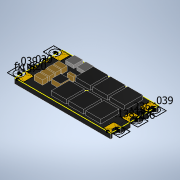
# Autodesk Inventor part: Circuit Board
Saved by Autodesk Inventor 2022 (Build 260153000, 153)
## iProperties
Created: 2022-09-18
Part Number: Circuit Board
Material: PPS Plastic
Document SubType Name: Modeling
Designer: Nathan Cai
Density: 1.637 g/cm^3
Appearance: Smooth - Black
Author: Nathan Cai
Autodesk Inventor part; units mm, degrees
ref_plane "YZ Plane" through (0, 0, 0) normal (1, 0, 0) x (0, 1, 0)
ref_plane "XZ Plane" through (0, 0, 0) normal (0, 1, 0) x (-1, 0, 0)
ref_plane "XY Plane" through (0, 0, 0) normal (0, 0, 1) x (1, 0, 0)
sketch "Sketch1" plane through (0, 0, 0) normal (0, 1, 0) x (-1, 0, 0)
  line L0 (-16, 8) -> (16, 8)
  line L1 (16, 8) -> (16, -8)
  line L2 (16, -8) -> (-16, -8)
  line L3 (-16, -8) -> (-16, 8)
  line L4 (-16, 8) -> (16, -8) construction
  line L5 (16, 8) -> (-16, -8) construction
  point P0 (0, 0)
  dimension "d0" = 32
  dimension "d1" = 16
  constraints: 12 end point, 2 midpoint, 2 parallel, 1 horizontal, 1 perpendicular
  measures "d0" distance of L1.end L2.end
  measures "d1" distance of L0.end L1.end
extrude "Extrusion1" add sketch "Sketch1" along normal blind 0.875
sketch "Sketch2" plane through (0, 0.875, 0) normal (0, 1, 0) x (1, 0, 0)
  line L0 (15, -8.0096) -> (15, 8) construction
  line L1 (16, 8) -> (-16, 8) projected
  line L2 (16, -8) -> (16, 8) projected
  circle A0 centre (16.5, 0) radius 1.5
  line L3 (-16, 8) -> (-16, -8) projected
  line L4 (-16, 0) -> (16, 0) construction
  circle A1 centre (16.5, 6) radius 1.5
  line L5 (18.75, -1.75) -> (13.25, -1.75)
  line L6 (13.25, -1.75) -> (13.25, 1.75)
  line L7 (13.25, 1.75) -> (18.75, 1.75)
  line L8 (18.75, 1.75) -> (18.75, -1.75)
  line L9 (18.75, -1.75) -> (13.25, 1.75) construction
  line L10 (13.25, -1.75) -> (18.75, 1.75) construction
  line L11 (13.25, 4.25) -> (13.25, 7.75)
  line L12 (18.75, 4.25) -> (13.25, 4.25)
  line L13 (18.75, 7.75) -> (18.75, 4.25)
  line L14 (18.75, 4.25) -> (13.25, 7.75) construction
  line L15 (13.25, 4.25) -> (18.75, 7.75) construction
  line L16 (13.25, 7.75) -> (18.75, 7.75)
  circle A2 centre (16.5, -6) radius 1.5
  line L17 (13.25, -4.25) -> (13.25, -7.75)
  line L18 (18.75, -4.25) -> (13.25, -4.25)
  line L19 (18.75, -7.75) -> (18.75, -4.25)
  line L20 (18.75, -4.25) -> (13.25, -7.75) construction
  line L21 (13.25, -4.25) -> (18.75, -7.75) construction
  line L22 (13.25, -7.75) -> (18.75, -7.75)
  line L23 (-16, -8) -> (16, -8) projected
  line L24 (0, -8) -> (0, 8) construction
  line L25 (-15, -8.0096) -> (-15, 8) construction
  circle A3 centre (-16.5, 6) radius 1.5
  line L26 (-13.25, 4.25) -> (-13.25, 7.75)
  line L27 (-18.75, 4.25) -> (-13.25, 4.25)
  line L28 (-18.75, 7.75) -> (-18.75, 4.25)
  line L29 (-18.75, 4.25) -> (-13.25, 7.75) construction
  line L30 (-13.25, 4.25) -> (-18.75, 7.75) construction
  line L31 (-13.25, 7.75) -> (-18.75, 7.75)
  line L32 (-13.25, -4.25) -> (-13.25, -7.75)
  line L33 (-18.75, -4.25) -> (-13.25, -4.25)
  line L34 (-18.75, -4.25) -> (-13.25, -7.75) construction
  line L35 (-13.25, -4.25) -> (-18.75, -7.75) construction
  line L36 (-13.25, -7.75) -> (-18.75, -7.75)
  line L37 (-18.75, -7.75) -> (-18.75, -4.25)
  circle A4 centre (-16.5, -6) radius 1.5
  circle A5 centre (-16, -2) radius 0.5
  circle A6 centre (-16, 2) radius 0.5
  circle A7 centre (-16, -2) radius 1
  circle A8 centre (-16, 2) radius 1
  point P0 (0, 0)
  point P1 (16, 6)
  point P2 (15, -8)
  point P3 (16, -6)
  point P4 (-16, 6)
  point P5 (-15, -8)
  point P6 (-16, -6)
  point P7 (-16, 4.5858)
  point P8 (-16, 7.4142)
  point P9 (16, 4.25)
  point P10 (16, 4.5858)
  point P11 (16, 7.4142)
  point P12 (16, 7.75)
  point P13 (16, -1.75)
  point P14 (16, -1.4142)
  point P15 (16, 1.4142)
  point P16 (16, 1.75)
  point P17 (16, -7.75)
  point P18 (16, -7.4142)
  point P19 (16, -4.5858)
  point P20 (16, -4.25)
  point P21 (-16, 7.75)
  point P22 (-16, 4.25)
  point P23 (-16, -4.25)
  point P24 (-16, -4.5858)
  point P25 (-16, -7.4142)
  point P26 (-16, -7.75)
  point P27 (-16, 3)
  point P28 (-16, 2.5)
  point P29 (-16, 1.5)
  point P30 (-16, 1)
  point P31 (-16, -1)
  point P32 (-16, -1.5)
  point P33 (-16, -2.5)
  point P34 (-16, -3)
  dimension "d4" = 1
  dimension "d5" = 3
  dimension "d8" = 6
  dimension "d13" = 5.5
  dimension "d14" = 3.5
  dimension "d17" = 6
  dimension "d22" = 1
  dimension "d23" = 4
  dimension "d28" = 0.5
  dimension "d29" = 0.5
  constraints: 68 end point, 26 symmetric about line, 14 midpoint, 9 centre point, 3 point on line, 3 vertical, 2 parallel, 1 horizontal, 1 perpendicular, 1 tangent, 18 other
  measures "d4" distance between parallel lines of L2 L0
  measures "d5" diameter of A0
  measures "d8" distance of A0.centre A1.centre
  measures "d13" distance of L6.end L7.end
  measures "d14" distance of L5.end L6.end
  measures "d17" distance of L6.end L11.end
  measures "d22" diameter of A5
  measures "d23" vertical distance of A4.centre A5.centre
  measures "d28" radial gap between concentric circles of A5 A7
  measures "d29" radial gap between concentric circles of A6 A8
extrude "Extrusion2" cut sketch "Sketch2" against normal through all contours A1 L2 | L2 A1 | A3 L3 | L3 A3 | A0 L2 | L2 A0 | A6 L3 | L3 A6 | A5 L3 | L3 A5 | A2 L2 | L2 A2 | A4 L3 | L3 A4
extrude "Extrusion3" add sketch "Sketch2" along normal blind 0.01 contours L2 A1 L12 L11 L16 | L31 L26 L27 L3 A3 | L2 A0 L5 L6 L7 | A8 L3 A6 | A7 L3 A5 | L2 A2 L22 L17 L18 | L33 L32 L36 L3 A4 picked at (-15.1792, 1.8887) picked at (-15.1792, -2.1113)
mirror "Mirror1" about plane through (0, 0, 0) normal (0, -1, 0) of "Extrusion1", "Extrusion2", "Extrusion3"
sketch "Sketch3" plane through (0, 0.875, 0) normal (0, 1, 0) x (1, 0, 0)
  line L0 (6.75, -1) -> (11.75, -1)
  line L1 (11.75, -1) -> (11.75, -7)
  line L2 (11.75, -7) -> (6.75, -7)
  line L3 (6.75, -7) -> (6.75, -1)
  line L4 (6.75, -1) -> (11.75, -7) construction
  line L5 (11.75, -1) -> (6.75, -7) construction
  line L6 (16, -4.25) -> (16, -1.75) projected
  line L7 (-16, -8) -> (16, -8) projected
  arc A0 (16, 1.4142) -> (16, -1.4142) centre (16.5, 0) ccw projected
  line L8 (-16, 0) -> (16.5, 0) construction
  line L9 (1, -1) -> (6, -1)
  line L10 (6, -1) -> (6, -7)
  line L11 (6, -7) -> (1, -7)
  line L12 (1, -7) -> (1, -1)
  line L13 (1, -1) -> (6, -7) construction
  line L14 (6, -1) -> (1, -7) construction
  line L15 (-4.75, -1) -> (0.25, -1)
  line L16 (0.25, -1) -> (0.25, -7)
  line L17 (0.25, -7) -> (-4.75, -7)
  line L18 (-4.75, -7) -> (-4.75, -1)
  line L19 (-4.75, -1) -> (0.25, -7) construction
  line L20 (0.25, -1) -> (-4.75, -7) construction
  line L21 (6.75, 1) -> (11.75, 1)
  line L22 (11.75, 1) -> (11.75, 7)
  line L23 (11.75, 7) -> (6.75, 7)
  line L24 (6.75, 7) -> (6.75, 1)
  line L25 (6.75, 1) -> (11.75, 7) construction
  line L26 (11.75, 1) -> (6.75, 7) construction
  line L27 (1, 1) -> (6, 1)
  line L28 (6, 1) -> (6, 7)
  line L29 (6, 7) -> (1, 7)
  line L30 (1, 7) -> (1, 1)
  line L31 (1, 1) -> (6, 7) construction
  line L32 (6, 1) -> (1, 7) construction
  line L33 (-4.75, 1) -> (0.25, 1)
  line L34 (0.25, 1) -> (0.25, 7)
  line L35 (0.25, 7) -> (-4.75, 7)
  line L36 (-4.75, 7) -> (-4.75, 1)
  line L37 (-4.75, 1) -> (0.25, 7) construction
  line L38 (0.25, 1) -> (-4.75, 7) construction
  point P0 (0, 0)
  point P1 (9.25, -4)
  point P2 (3.5, -4)
  point P3 (-2.25, -4)
  point P4 (9.25, 4)
  point P5 (3.5, 4)
  point P6 (-2.25, 4)
  dimension "d30" = 5
  dimension "d31" = 6
  dimension "d32" = 4.25
  dimension "d33" = 1
  dimension "d36" = 5.75
  constraints: 74 end point, 15 symmetric about line, 12 midpoint, 3 horizontal, 2 parallel, 1 perpendicular, 22 other
  measures "d30" distance of L1.end L2.end
  measures "d31" distance of L0.end L1.end
  measures "d32" distance between parallel lines of L6 L1
  measures "d33" distance between parallel lines of L7 L2
  measures "d36" distance of L0.start L9.start
extrude "Extrusion4" add sketch "Sketch3" along normal blind 1.35
sketch "Sketch4" plane through (0, 0.875, 0) normal (0, 1, 0) x (1, 0, 0)
  line L0 (-11.5, 7.5) -> (-8.75, 7.5)
  line L1 (-8.75, 7.5) -> (-8.75, 4.5)
  line L2 (-8.75, 4.5) -> (-11.5, 4.5)
  line L3 (-11.5, 4.5) -> (-11.5, 7.5)
  line L4 (-11.5, 7.5) -> (-8.75, 4.5) construction
  line L5 (-8.75, 7.5) -> (-11.5, 4.5) construction
  line L6 (16, 8) -> (-16, 8) projected
  line L7 (-16, 4.25) -> (-16, 3) projected
  line L8 (-7.75, 7.5) -> (-5, 7.5)
  line L9 (-5, 7.5) -> (-5, 4.5)
  line L10 (-5, 4.5) -> (-7.75, 4.5)
  line L11 (-7.75, 4.5) -> (-7.75, 7.5)
  line L12 (-7.75, 7.5) -> (-5, 4.5) construction
  line L13 (-5, 7.5) -> (-7.75, 4.5) construction
  point P0 (0, 0)
  point P1 (-10.125, 6)
  point P2 (-6.375, 6)
  dimension "d43" = 2.75
  dimension "d44" = 3
  dimension "d45" = 0.5
  dimension "d46" = 4.5
  dimension "d49" = 3.75
  constraints: 24 end point, 4 midpoint, 2 horizontal, 2 parallel, 1 collinear, 1 perpendicular, 10 other
  measures "d43" distance of L1.end L2.end
  measures "d44" distance of L0.end L1.end
  measures "d45" distance between parallel lines of L6 L0
  measures "d46" distance between parallel lines of L7 L3
  measures "d49" distance of L0.start L8.start
extrude "Extrusion5" add sketch "Sketch4" along normal blind 1
sketch "Sketch5" plane through (0, 0.875, 0) normal (0, 1, 0) x (1, 0, 0)
  line L0 (-12, 2.7) -> (-9.15, 2.7)
  line L1 (-9.15, 2.7) -> (-9.15, 0.95)
  line L2 (-9.15, 0.95) -> (-12, 0.95)
  line L3 (-12, 0.95) -> (-12, 2.7)
  line L4 (-12, 2.7) -> (-9.15, 0.95) construction
  line L5 (-9.15, 2.7) -> (-12, 0.95) construction
  line L6 (-12, 0.55) -> (-9.15, 0.55)
  line L7 (-9.15, 0.55) -> (-9.15, -1.2)
  line L8 (-9.15, -1.2) -> (-12, -1.2)
  line L9 (-12, -1.2) -> (-12, 0.55)
  line L10 (-12, 0.55) -> (-9.15, -1.2) construction
  line L11 (-9.15, 0.55) -> (-12, -1.2) construction
  line L12 (-12, -1.6) -> (-9.15, -1.6)
  line L13 (-9.15, -1.6) -> (-9.15, -3.35)
  line L14 (-9.15, -3.35) -> (-12, -3.35)
  line L15 (-12, -3.35) -> (-12, -1.6)
  line L16 (-12, -1.6) -> (-9.15, -3.35) construction
  line L17 (-9.15, -1.6) -> (-12, -3.35) construction
  line L18 (-12, -3.75) -> (-9.15, -3.75)
  line L19 (-9.15, -3.75) -> (-9.15, -5.5)
  line L20 (-9.15, -5.5) -> (-12, -5.5)
  line L21 (-12, -5.5) -> (-12, -3.75)
  line L22 (-12, -3.75) -> (-9.15, -5.5) construction
  line L23 (-9.15, -3.75) -> (-12, -5.5) construction
  line L24 (-16, -8) -> (16, -8) projected
  line L25 (-16, -3) -> (-16, -4.25) projected
  line L26 (-8, -3.65) -> (-5, -3.65)
  line L27 (-5, -3.65) -> (-5, -0.65)
  line L28 (-5, -0.65) -> (-8, -0.65)
  line L29 (-8, -0.65) -> (-8, -3.65)
  line L30 (-8, -3.65) -> (-5, -0.65) construction
  line L31 (-5, -3.65) -> (-8, -0.65) construction
  line L32 (-7, 1.5) -> (-5, 1.5)
  line L33 (-5, 1.5) -> (-5, 0.5)
  line L34 (-5, 0.5) -> (-7, 0.5)
  line L35 (-7, 0.5) -> (-7, 1.5)
  line L36 (-7, 1.5) -> (-5, 0.5) construction
  line L37 (-5, 1.5) -> (-7, 0.5) construction
  point P0 (0, 0)
  point P1 (-10.575, 1.825)
  point P2 (-10.575, -0.325)
  point P3 (-10.575, -2.475)
  point P4 (-10.575, -4.625)
  point P5 (-6.5, -2.15)
  point P6 (-6, 1)
  dimension "d56" = 2.85
  dimension "d57" = 1.75
  dimension "d60" = 2.15
  dimension "d65" = 2.5
  dimension "d66" = 4
  dimension "d67" = 3
  dimension "d68" = 3
  dimension "d69" = 4.35
  dimension "d70" = 8
  dimension "d71" = 2
  dimension "d72" = 1
  dimension "d73" = 9
  dimension "d74" = 8.5
  constraints: 72 end point, 12 midpoint, 6 parallel, 3 horizontal, 3 perpendicular, 1 collinear, 1 vertical, 32 other
  measures "d56" distance of L1.end L2.end
  measures "d57" distance of L0.end L1.end
  measures "d60" distance of L0.start L6.start
  measures "d65" distance between parallel lines of L24 L20
  measures "d66" distance between parallel lines of L25 L21
  measures "d67" distance of L28.end L27.end
  measures "d68" distance of L27.end L26.end
  measures "d69" distance between parallel lines of L24 L26
  measures "d70" distance between parallel lines of L25 L29
  measures "d71" distance of L33.end L34.end
  measures "d72" distance of L32.end L33.end
  measures "d73" distance between parallel lines of L25 L35
  measures "d74" distance between parallel lines of L24 L34
extrude "Extrusion6" add sketch "Sketch5" along normal blind 1.5
equation "\"d28\" = d29"
body "Solid1"
